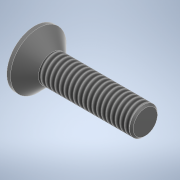
# Autodesk Inventor part: M3 x 10 mm FHCS
Saved by Autodesk Inventor 2022 (Build 260153000, 153)
## iProperties
Created: 2022-03-21
Part Number: M3 x 10 mm FHCS
Material: Generic
Document SubType Name: Modeling
Designer: Nick
Density: 1 g/cm^3
Appearance: Smooth - Black
Author: Nick
Autodesk Inventor part; units mm, degrees
ref_plane "YZ Plane" through (0, 0, 0) normal (1, 0, 0) x (0, 1, 0)
ref_plane "XZ Plane" through (0, 0, 0) normal (0, 1, 0) x (-1, 0, 0)
ref_plane "XY Plane" through (0, 0, 0) normal (0, 0, 1) x (1, 0, 0)
sketch "Sketch1" plane through (0, 0, 0) normal (0, 0, 1) x (1, 0, 0)
  line L0 (0, 0) -> (0, 3)
  line L1 (0, 3) -> (0.4, 3)
  line L2 (0.4, 3) -> (1.9, 1.5)
  line L3 (1.9, 1.5) -> (11.9, 1.5)
  line L4 (11.9, 1.5) -> (11.9, 0)
  line L5 (11.9, 0) -> (0, 0)
  dimension "d0" = 10
  dimension "d1" = 45
  dimension "d2" = 1.9
  dimension "d3" = 1.5
  dimension "d4" = 3
  constraints: 12 end point, 3 perpendicular, 1 parallel, 1 vertical
  measures "d0" distance of L2.end L3.end
  measures "d1" angle of L5 L2
  measures "d2" distance from line of L2.end L0
  measures "d3" distance of L3.end L4.end
  measures "d4" distance between parallel lines of L5 L1
revolve "Revolution1" add sketch "Sketch1" angle 360 about axis through (11.9, 0, 0) along (-1, 0, 0)
sketch "Sketch2" plane through (0, 0, 0) normal (-1, 0, 0) x (0, 0, 1)
  line L0 (0.5725, -1.0028) -> (-0.5822, -0.9972)
  line L1 (-0.5822, -0.9972) -> (-1.1547, 0.0056)
  line L2 (-1.1547, 0.0056) -> (-0.5725, 1.0028)
  line L3 (-0.5725, 1.0028) -> (0.5822, 0.9972)
  line L4 (0.5822, 0.9972) -> (1.1547, -0.0056)
  line L5 (1.1547, -0.0056) -> (0.5725, -1.0028)
  point P0 (0, 0)
  point P1 (0, 0)
  dimension "d6" = 2
  constraints: 12 end point, 1 coincident, 13 other
  measures "d6" distance between parallel lines of L0 L3
extrude "Extrusion1" cut sketch "Sketch2" against normal blind 1.2
thread "Thread1" size "M3x0.5" class "6g" standard "ANSI Metric M Profile" full length
chamfer "Chamfer1" distance 0.2 angle 45 1 edges at (11.9, -1.5, 0)
body "Solid1"
